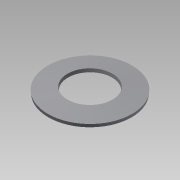
# Autodesk Inventor part: Partspring
Saved by Autodesk Inventor 2014 (Build 180170000, 170)
## iProperties
Created: 2016-03-22
Part Number: Partspring
Material: Silver
Document SubType Name: Modeling
Designer: admin
Density: 1 g/cm^3
Appearance: Silver
Author: admin
Autodesk Inventor part; units mm, degrees
ref_plane "YZ Plane" through (0, 0, 0) normal (1, 0, 0) x (0, 1, 0)
ref_plane "XZ Plane" through (0, 0, 0) normal (0, 1, 0) x (-1, 0, 0)
ref_plane "XY Plane" through (0, 0, 0) normal (0, 0, 1) x (1, 0, 0)
sketch "Sketch1" plane through (0, 0, 0) normal (0, 1, 0) x (-1, 0, 0)
  line L0 (-7.813, 1.5707) -> (-5.9534, 1.8234)
  line L1 (-5.9534, 1.8234) -> (-5.9938, 2.1207)
  line L2 (-5.9938, 2.1207) -> (-7.8534, 1.8679)
  line L3 (-7.8534, 1.8679) -> (-7.813, 1.5707)
  line L4 (-3.8534, 0) -> (-3.8534, 5.7761)
  point P0 (0, 0)
  dimension "d2" = 0.3
  dimension "d3" = 0.55
  dimension "d4" = 4
  dimension "d5" = 2.1
  constraints: 10 end point, 2 parallel, 1 perpendicular, 1 vertical
  measures "d2" distance between parallel lines of L0 L2
  measures "d3" vertical distance of L1.end L0.start
  measures "d4" distance from line of L4 L2.end
  measures "d5" distance from line of L4 L0.end
revolve "Revolution1" add sketch "Sketch1" angle 360 about axis through (3.8534, 0, 0) along (0, 0, 1)
body "Solid1"
